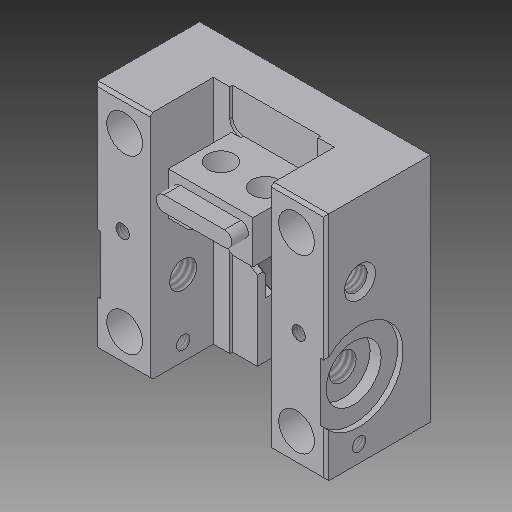
# Autodesk Inventor part: Support coulisse
Saved by Autodesk Inventor 2017 (Build 210142000, 142)
## iProperties
Company: FABLAB Frenchmakers
Part Number: Support coulisse
Material: ----------
Document SubType Name: Modeling
Designer: FABLAB Frenchmakers
Density: 7.86 g/cm^3
Appearance: Métal - Acier
Mass: 122.678 g
Surface Area: 102.295 cm^2
Volume: 15.6079 cm^3
Project: 1420 Vauban 3D XL
Catalog Web Link: http://frenchmakers.com/
Stock Number: 1420-05-14
Autodesk Inventor part; units mm, degrees
note: some values were not read from the file. Chosen so that the rebuilt part matches the saved one: direction of "Perçage7".
ref_plane "YZ Plane" through (0, 0, 0) normal (1, 0, 0) x (0, 1, 0)
ref_plane "XZ Plane" through (0, 0, 0) normal (0, 1, 0) x (-1, 0, 0)
ref_plane "XY Plane" through (0, 0, 0) normal (0, 0, 1) x (1, 0, 0)
sketch "Esquisse1" plane through (0, 0, 0) normal (0, 0, 1) x (1, 0, 0)
  line L0 (-21, -21) -> (21, -21)
  line L1 (21, -21) -> (21, 21)
  line L2 (21, 21) -> (-21, 21)
  line L3 (-21, 21) -> (-21, -21)
  line L4 (-21, -21) -> (21, 21) construction
  line L5 (21, -21) -> (-21, 21) construction
  point P0 (0, 0)
  dimension "d0" = 42
  dimension "d1" = 42
  constraints: 12 end point, 2 midpoint, 2 parallel, 1 horizontal, 1 perpendicular
  measures "d0" distance of L2.end L1.end
  measures "d1" distance of L1.end L0.end
extrude "Extrusion1" add sketch "Esquisse1" along normal blind 19.5
sketch "Esquisse2" plane through (0, 0, 19.5) normal (0, 0, 1) x (1, 0, 0)
  line L0 (-11, -21) -> (11, -21)
  line L1 (11, -21) -> (11, 21)
  line L2 (11, 21) -> (-11, 21)
  line L3 (-11, 21) -> (-11, -21)
  line L4 (-11, -21) -> (11, 21) construction
  line L5 (11, -21) -> (-11, 21) construction
  line L6 (21, 21) -> (-21, 21) projected
  point P0 (0, 0)
  dimension "d4" = 22
  constraints: 12 end point, 2 midpoint, 2 parallel, 1 collinear, 1 horizontal, 1 perpendicular
  measures "d4" distance between parallel lines of L3 L1
extrude "Extrusion2" cut sketch "Esquisse2" against normal blind 11.5
sketch "Esquisse3" plane through (0, 0, 19.5) normal (0, 0, 1) x (1, 0, 0)
  line L0 (11, -21) -> (21, -21) projected
  line L1 (21, -21) -> (21, 21) projected
  point P0 (0, 0)
  point P1 (-15.625, -15.625)
  point P2 (-15.625, 15.625)
  point P3 (15.625, 15.625)
  point P4 (15.625, -15.625)
  dimension "d7" = 31.25
  dimension "d8" = 31.25
  dimension "d109" = 15.625
  dimension "d110" = 15.625
  constraints: 2 horizontal alignment, 2 vertical alignment
  measures "d7" distance of point (15.625, 15.625) point (-15.625, 15.625)
  measures "d8" distance of point (15.625, -15.625) point (15.625, 15.625)
  measures "d109" horizontal distance of point (0, 0) point (-15.625, 15.625)
  measures "d110" horizontal distance of point (15.625, -15.625) point (0, 0)
hole "Perçage1" at (-15.625, -15.625, 19.5) at (-15.625, 15.625, 19.5) at (15.625, 15.625, 19.5) at (15.625, -15.625, 19.5) direction (0, 0, -1) diameter 3.3 end through all counterbore diameter 6.5 counterbore depth 13.6
sketch "Esquisse11" plane through (21, -21, 0) normal (1, 0, 0) x (0, 0, -1)
  line L0 (0, 42) -> (-19.5, 42) projected
  line L1 (-19.5, 0) -> (-19.5, 42) projected
  point P0 (0, 21)
  point P1 (-13.35, 28.5)
  dimension "d67" = 13.5
  dimension "d68" = 6.15
  measures "d67" distance from line of L0 point (-13.35, 28.5)
  measures "d68" distance from line of L1 point (-13.35, 28.5)
hole "Perçage6" at (21, 7.5, 13.35) direction (-1, 0, 0) diameter 4.134 end through all thread size "M5x0.8" class "6H" standard "ISO Metric profile"
sketch "Esquisse4" plane through (0, 0, 8) normal (0, 0, 1) x (1, 0, 0)
  line L0 (-7.7, 14) -> (7.7, 14)
  line L1 (7.7, 14) -> (7.7, 6.25)
  line L2 (7.7, 6.25) -> (-7.7, 6.25)
  line L3 (-7.7, 6.25) -> (-7.7, 14)
  line L4 (-7.7, 14) -> (7.7, 6.25) construction
  line L5 (7.7, 14) -> (-7.7, 6.25) construction
  line L6 (21, 21) -> (11, 21) projected
  point P0 (0, 0)
  point P1 (0, 10.125)
  point P2 (0, 10.125)
  dimension "d18" = 7.75
  dimension "d19" = 15.4
  dimension "d20" = 7
  constraints: 12 end point, 3 midpoint, 2 parallel, 1 horizontal, 1 perpendicular, 1 vertical alignment
  measures "d18" distance between parallel lines of L2 L0
  measures "d19" distance of L1.end L2.end
  measures "d20" distance between parallel lines of L6 L0
extrude "Extrusion3" add sketch "Esquisse4" along normal blind 11.5
sketch "Esquisse5" plane through (0, 0, 19.5) normal (0, 0, 1) x (1, 0, 0)
  line L0 (-5.5, 11.125) -> (5.5, 11.125) construction
  line L1 (-5.5, 9.75) -> (5.5, 9.75)
  line L2 (5.5, 12.5) -> (-5.5, 12.5)
  arc A0 (-5.5, 12.5) -> (-5.5, 9.75) centre (-5.5, 11.125) ccw
  arc A1 (5.5, 9.75) -> (5.5, 12.5) centre (5.5, 11.125) ccw
  line L3 (-7.7, 14) -> (7.7, 14) projected
  point P0 (0, 0)
  point P1 (0, 11.125)
  dimension "d24" = 2.75
  dimension "d25" = 13.75
  dimension "d26" = 1.5
  constraints: 8 end point, 4 point on circle, 4 tangent, 2 centre point, 1 horizontal, 1 midpoint, 1 parallel, 1 vertical alignment
  measures "d24" distance between parallel lines of L1 L2
  measures "d26" distance between parallel lines of L3 L2
extrude "Extrusion4" add sketch "Esquisse5" along normal blind 3
sketch "Esquisse6" plane through (-7.7, 14, 8) normal (0, 1, 0) x (1, 0, 0)
  line L0 (15.4, -11.5) -> (0, -11.5) projected
  point P0 (7.7, 8)
  point P1 (11.725, -5.6)
  point P2 (3.675, -5.6)
  dimension "d29" = 8.05
  dimension "d30" = 5.9
  dimension "d31" = 4.025
  constraints: 1 horizontal alignment
  measures "d29" distance of point (3.675, -5.6) point (11.725, -5.6)
  measures "d30" distance from line of L0 point (3.675, -5.6)
  measures "d31" horizontal distance of point (7.7, 8) point (3.675, -5.6)
hole "Perçage2" at (4.025, 14, 13.6) at (-4.025, 14, 13.6) direction (0, -1, 0) diameter 4.85 depth 5.8
sketch "Esquisse7" plane through (0, 0, 0) normal (0, 0, -1) x (-1, 0, 0)
  point P0 (0, 0)
  point P1 (0, 0)
  constraints: 1 coincident
hole "Perçage3" at (0, 0, 0) direction (0, 0, 1) diameter 23 depth 6 counterbore diameter 36.5 counterbore depth 4
sketch "Esquisse8" plane through (0, 0, 6) normal (0, 0, -1) x (-1, 0, 0)
  point P0 (0, 0)
  point P1 (0, 0)
  constraints: 1 coincident
hole "Perçage4" at (0, 0, 6) direction (0, 0, 1) diameter 15 end through all
sketch "Esquisse9" plane through (0, 0, 8) normal (0, 0, 1) x (1, 0, 0)
  line L0 (-3.5, -21) -> (3.5, -21)
  line L1 (3.5, -21) -> (3.5, 0)
  line L2 (3.5, 0) -> (-3.5, 0)
  line L3 (-3.5, 0) -> (-3.5, -21)
  line L4 (11, -21) -> (-11, -21) projected
  point P0 (0, 0)
  dimension "d53" = 7
  dimension "d54" = 3.5
  constraints: 8 end point, 2 parallel, 1 collinear, 1 horizontal, 1 midpoint, 1 perpendicular
  measures "d53" distance between parallel lines of L1 L3
  measures "d54" distance from line of point (0, 0) L1
extrude "Extrusion5" cut sketch "Esquisse9" against normal blind 4.5
sketch "Esquisse10" plane through (0, 0, 19.5) normal (0, 0, 1) x (1, 0, 0)
  line L0 (11, -21) -> (21, -21) projected
  point P0 (0, 0)
  point P1 (-16, 0)
  point P2 (16, 0)
  dimension "d57" = 32
  dimension "d58" = 16
  dimension "d59" = 21
  constraints: 1 horizontal alignment
  measures "d57" distance of point (16, 0) point (-16, 0)
  measures "d58" distance of point (0, 0) point (16, 0)
  measures "d59" distance from line of L0 point (16, 0)
hole "Perçage5" at (-16, 0, 19.5) at (16, 0, 19.5) direction (0, 0, -1) diameter 2.459 end through all thread size "M3x0.5" class "6H" standard "ISO Metric profile"
sketch "Esquisse12" plane through (21, -21, 0) normal (1, 0, 0) x (0, 0, -1)
  circle A0 centre (-13.5, 13.7) radius 8
  line L0 (0, 0) -> (-19.5, 0) projected
  line L1 (0, 0) -> (0, 42) projected
  point P0 (0, 21)
  dimension "d76" = 16
  dimension "d77" = 13.7
  dimension "d78" = 13.5
  constraints: 1 centre point, 1 coincident
  measures "d76" diameter of A0
  measures "d77" distance from line of L0 A0.centre
  measures "d78" distance from line of L1 A0.centre
extrude "Extrusion6" cut sketch "Esquisse12" against normal blind 1
sketch "Esquisse13" plane through (20, -21, 0) normal (1, 0, 0) x (0, 0, -1)
  line L0 (-19.5, 8.4085) -> (-19.5, 18.9915) construction
  arc A0 (-19.5, 8.4085) -> (-19.5, 18.9915) centre (-13.5, 13.7) ccw construction
  point P0 (0, 21)
  constraints: 1 coincident
hole "Perçage7" at (20, -7.3, 13.5) direction (-1, 0, 0) diameter 4.917 end up to surface counterbore diameter 10 counterbore depth 2 thread size "M6x1" class "6H" standard "ISO Metric profile"
mirror "Symétrie1" about plane through (0, 0, 0) normal (1, 0, 0) of "Extrusion6", "Perçage7"
chamfer "Chanfrein1" distance 0.75 angle 45 2 edges at (21, 7.5, 15.417) (-21, 7.5, 15.417)
sketch "Esquisse14" plane through (-21, -21, 0) normal (-1, 0, 0) x (0, 0, 1)
  line L0 (19.5, 8.4085) -> (19.5, 0) projected
  circle A0 centre (13.5, 13.7) radius 2.4585 construction
  line L1 (0, 0) -> (19.5, 0) projected
  point P0 (0, 21)
  point P1 (13.5, 3.011)
  dimension "d92" = 3.011
  constraints: 1 vertical alignment
  measures "d92" distance from line of L1 point (13.5, 3.011)
hole "Perçage8" at (-21, -17.989, 13.5) direction (1, 0, 0) diameter 2.459 end through all thread size "M3x0.5" class "6H" standard "ISO Metric profile"
chamfer "Chanfrein2" distance 0.5 angle 45 15 edges at (-16, 21, 19.5) (-21, 9.4958, 19.5) (-16, -21, 19.5) (-21, -16.7958, 19.5) (16, -21, 19.5) (21, -16.7958, 19.5) (21, 9.4958, 19.5) (16, 21, 19.5) (0, -21, 0) (-21, 0, 0) (21, 0, 0) (0, 21, 0) (0, -18.25, 0) (0, 11.5, 4) (0, 7.5, 6)
sketch "Esquisse15" plane through (0, 0, 8) normal (0, 0, 1) x (1, 0, 0)
  line L0 (-8, -21) -> (8, -21)
  line L1 (8, -21) -> (8, 4.25)
  line L2 (6, 6.25) -> (-6, 6.25)
  line L3 (-8, 4.25) -> (-8, -21)
  line L4 (3.5, -21) -> (-3.5, -21) projected
  line L5 (4.1458, 6.25) -> (7.7, 6.25) projected
  line L6 (-8, 21) -> (8, 21)
  line L7 (8, 21) -> (8, 16)
  line L8 (6, 14) -> (-6, 14)
  line L9 (-8, 16) -> (-8, 21)
  line L10 (7.7, 14) -> (-7.7, 14) projected
  line L11 (-11, 21) -> (11, 21) projected
  arc A0 (-6, 6.25) -> (-8, 4.25) centre (-6, 4.25) ccw
  arc A1 (8, 4.25) -> (6, 6.25) centre (6, 4.25) ccw
  arc A2 (-8, 16) -> (-6, 14) centre (-6, 16) ccw
  arc A3 (6, 14) -> (8, 16) centre (6, 16) ccw
  point P0 (0, 0)
  dimension "d103" = 16
  dimension "d104" = 8
  dimension "d106" = 2
  constraints: 16 end point, 8 point on circle, 8 tangent, 6 collinear, 4 centre point, 4 parallel, 3 equal radius, 2 horizontal, 2 perpendicular
  measures "d103" distance between parallel lines of L1 L3
  measures "d104" distance from line of point (0, 0) L1
  measures "d106" radius of A0
extrude "Extrusion7" cut sketch "Esquisse15" against normal blind 0.5
equation "\"d8\" = d7"
equation "\"d109\" = 0.5 * d7"
equation "\"d110\" = 0.5 * d7"
equation "\"d31\" = 0.5 * d29"
equation "\"d54\" = 0.5 * d53"
equation "\"d58\" = 0.5 * d57"
equation "\"d104\" = 0.5 * d103"
